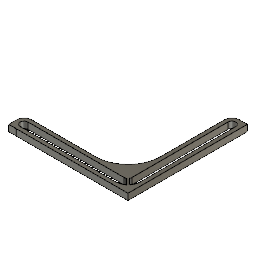
lidar_camera_frontplate v1 (Autodesk Fusion 360 archive; units mm, degrees)
design "front_L"
Autodesk Fusion 360 part; units mm, degrees
note: some values were not read from the file. Chosen so that the rebuilt part matches the saved one: that a step has no effect. Set by a fixed rule: which sketch regions a step uses.
sketch "Sketch1" plane through (0, 0, 0) normal (0, 0, 1) x (1, 0, 0)
  line L0 (20, 90) -> (17, 90)
  line L1 (17, 16) -> (17, 90)
  line L2 (23, 90) -> (23, 16)
  line L3 (-60, 7) -> (14, 7)
  line L4 (14, 13) -> (-60, 13)
  arc A0 (23, 90) -> (17, 89.9988) centre (20, 90) ccw
  arc A1 (-60, 13) -> (-60, 7) centre (-60, 10) ccw
  line L5 (-60, 4) -> (-66, 4)
  line L6 (-66, 4) -> (-66, 10)
  line L7 (-60, 16) -> (-11, 16)
  line L8 (14, 41) -> (14, 90)
  line L9 (20, 96) -> (26, 96)
  line L10 (26, 96) -> (26, 4)
  line L11 (26, 4) -> (-60, 4)
  arc A2 (-60, 16) -> (-66, 10) centre (-60, 10) ccw
  arc A3 (-11, 16) -> (14, 41) centre (-11, 41) ccw
  arc A4 (20, 96) -> (14, 90) centre (20, 90) ccw
  line L12 (18, 13) -> (16.823, 14.177)
  line L13 (18, 13) -> (20.4495, 10.5505)
  line L14 (17, 12) -> (15.823, 13.177)
  line L15 (17, 12) -> (19.8443, 9.1557)
  arc A5 (14, 13) -> (15.2595, 13.2772) centre (14, 16) ccw
  arc A6 (16.7228, 14.7405) -> (17, 16) centre (14, 16) ccw
  arc A7 (14, 7) -> (19.8443, 9.1557) centre (14, 16) ccw
  arc A8 (21.2032, 10.6043) -> (23, 16) centre (14, 16) ccw
  arc A9 (15.823, 13.177) -> (15.2595, 13.2772) centre (15.4695, 12.8234) ccw
  arc A10 (16.7228, 14.7405) -> (16.823, 14.177) centre (17.1766, 14.5305) ccw
  arc A11 (20.4495, 10.5505) -> (21.2032, 10.6043) centre (20.803, 10.9041) ccw
  dimension "d1" = 6
  dimension "d4" = 6
  dimension "d6" = 3
  dimension "d7" = 9
  dimension "d8" = 3
  dimension "d9" = 6
  dimension "d10" = 25
  dimension "d11" = 6
  dimension "d13" = 92
  dimension "d14" = 92
  dimension "d15" = 12
  dimension "d16" = 0.5
  constraint coincident L0.start A0.centre
  constraint coincident L0.end A0
  constraint horizontal L0
  constraint perpendicular L0 L1
  constraint tangent L4 A1
  constraint coincident L1 A0.end
  constraint tangent L1 A5
  constraint tangent L4 A5
  constraint horizontal L3
  constraint tangent L2 A7
  constraint tangent L3 A7
  constraint perpendicular L5 L6
  constraint perpendicular L7 L8
  constraint perpendicular L8 L9
  constraint perpendicular L9 L10
  constraint tangent L6 A2
  constraint tangent L7 A2
  constraint tangent L8 A3
  constraint tangent L7 A3
  constraint tangent L9 A4
  constraint tangent L8 A4
  constraint concentric A5 A6
  constraint concentric A7 A8
  constraint tangent L14 A9
  constraint tangent A5 A9
  constraint tangent L12 A10
  constraint tangent A6 A10
  constraint equal A9 A10
  constraint tangent L13 A11
  constraint tangent A8 A11
  constraint equal A9 A11
  measures "d1" diameter of A0
  measures "d4" diameter of A1
  measures "d6" radius of A5
  measures "d7" radius of A7
  measures "d8" distance of L3.start L5.start
  measures "d9" radius of A2
  measures "d10" radius of A3
  measures "d11" radius of A4
  measures "d13" distance of L9.end L10.end
  measures "d14" distance of L5.end L10.end
  measures "d15" distance of L7 L11
  measures "d16" radius of A9
extrude "Extrude1" add sketch "Sketch1" along normal blind 5

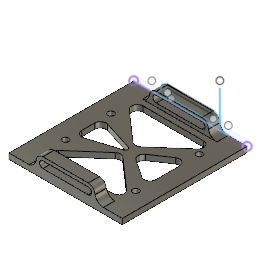
design "lidar_holder"
Autodesk Fusion 360 part; units mm, degrees
sketch "Sketch1" plane through (0, 0, 0) normal (0, 0, 1) x (1, 0, 0)
  line L0 (0, 0) -> (100, 0)
  line L1 (100, 0) -> (100, 110)
  line L2 (100, 110) -> (0, 110)
  line L3 (0, 110) -> (0, 0)
  circle A0 centre (15, 35) radius 2.75
  circle A1 centre (15, 75) radius 2.75
  circle A2 centre (85, 83) radius 2.75
  circle A3 centre (85, 27) radius 2.75
  line L4 (85, 35) -> (85, 75)
  line L5 (15, 67.5) -> (15, 42.5)
  line L6 (85, 35) -> (55, 55)
  line L7 (85, 75) -> (55, 55)
  line L8 (50, 50) -> (10, 15)
  line L9 (10, 15) -> (90, 15)
  line L10 (90, 15) -> (50, 50)
  line L11 (50, 60) -> (90, 95)
  line L12 (90, 95) -> (10, 95)
  line L13 (10, 95) -> (50, 60)
  line L14 (15, 42.5) -> (54.5, 55)
  line L15 (54.5, 55) -> (15, 67.5)
  dimension "d1" = 5.5
  dimension "d2" = 5.5
  dimension "d3" = 5.5
  dimension "d4" = 5.5
  dimension "d5" = 40
  dimension "d6" = 56
  dimension "d7" = 70
  dimension "d9" = 100
  dimension "d10" = 110
  dimension "d11" = 27
  dimension "d12" = 15
  dimension "d63" = 15
  dimension "d66" = 15
  dimension "d67" = 7.5
  dimension "d68" = 7.5
  dimension "d72" = 15
  dimension "d73" = 15
  dimension "d76" = 50
  dimension "d77" = 10
  dimension "d78" = 10
  dimension "d80" = 56.31
  dimension "d81" = 56.31
  dimension "d140" = 10
  dimension "d141" = 41.186
  dimension "d142" = 41.186
  dimension "d143" = 72.44
  dimension "d152" = 35
  dimension "d153" = 35
  dimension "d154" = 35
  constraint horizontal L0
  constraint vertical L1
  constraint horizontal L2
  constraint vertical L3
  constraint coincident L0.start L3.end
  constraint vertical A0.centre A1.centre
  constraint vertical A2.centre A3.centre
  constraint vertical L4
  constraint vertical L5
  constraint horizontal L9
  constraint parallel L8 L11
  constraint parallel L10 L13
  constraint horizontal L6.end L14.end
  measures "d1" diameter of A0
  measures "d2" diameter of A1
  measures "d3" diameter of A2
  measures "d4" diameter of A3
  measures "d5" vertical distance of A0.centre A1.centre
  measures "d6" vertical distance of A2.centre A3.centre
  measures "d7" horizontal distance of A1.centre A2.centre
  measures "d9" distance of L1.end L2.end
  measures "d10" distance of L0.end L1.end
  measures "d11" distance of L2 A2.centre
  measures "d12" distance of L1 A3.centre
  measures "d63" distance of L1 L4
  measures "d66" distance of L3 L5
  measures "d67" distance of A0.centre L5.end
  measures "d68" distance of A1.centre L5.start
  measures "d72" distance of L0 L9
  measures "d73" distance of L2 L12
  measures "d76" distance of L2 L11.start
  measures "d77" distance of L3 L12.end
  measures "d78" distance of L3 L8.end
  measures "d80" angle of L4 L6
  measures "d81" angle of L4 L7
  measures "d140" distance of L1 L9.end
  measures "d141" angle of L12 L13
  measures "d142" angle of L11 L12
  measures "d143" angle of L5 L14
  measures "d152" distance of L2 L4.end
  measures "d153" distance of L0 L4.start
  measures "d154" distance of L2 A1.centre
extrude "Extrude13" add sketch "Sketch1" along normal blind 5
sketch "Sketch2" plane through (0, 110, 0) normal (0, 1, 0) x (-1, 0, 0)
  line L0 (-100, 0) -> (0, 0)
  line L1 (0, 0) -> (0, 10)
  line L2 (0, 10) -> (-100, 10)
  line L3 (-100, 10) -> (-100, 0)
  arc A0 (-29.9676, 8) -> (-29.9676, 14) centre (-29.9676, 11) ccw
  line L4 (-75.9121, 43) -> (-76, 43)
  line L5 (-29.9676, 8) -> (-33.1608, 8)
  line L6 (-29.9676, 14) -> (-69.9676, 14)
  line L7 (-69.9676, 8) -> (-29.9676, 8)
  arc A1 (-69.9676, 17) -> (-75.9676, 11) centre (-69.9676, 11) ccw
  line L8 (-69.9676, 17) -> (-29.9676, 17)
  line L9 (-76, 37.0055) -> (-75.9676, 11)
  arc A2 (-69.9676, 14) -> (-69.9676, 8) centre (-69.9676, 11) ccw
  arc A3 (-23.9676, 11) -> (-29.9676, 17) centre (-29.9676, 11) ccw
  line L10 (-23.9676, 5) -> (-75.9676, 5)
  line L11 (-75.9676, 5) -> (-83.3383, 5)
  line L12 (-23.9676, 5) -> (-17.9511, 5)
  arc A4 (-83.3383, 5) -> (-75.9676, 11) centre (-83.3383, 12.5273) ccw
  arc A5 (-23.9676, 11) -> (-17.9511, 5) centre (-16.0025, 12.9705) ccw
  line L13 (0, 5) -> (-100, 5)
  dimension "d108" = 6
  dimension "d109" = 6
  dimension "d110" = 3
  dimension "d111" = 40
  dimension "d112" = 6
  dimension "d115" = 6
  dimension "d116" = 40
  dimension "d119" = 6
  dimension "d120" = 52
  dimension "d121" = 3
  dimension "d135" = 12
  constraint tangent L6 A2
  constraint horizontal L6
  constraint horizontal L8
  constraint parallel L4 L8
  constraint concentric A1 A2
  constraint tangent A1 L9
  constraint coincident L8.start A1
  constraint coincident L9.start A1
  constraint coincident A1.start L8
  constraint concentric A0 A3
  constraint tangent L11 A4
  constraint horizontal L10
  measures "d108" diameter of A2
  measures "d109" diameter of A0
  measures "d110" distance of L6 L8
  measures "d111" distance of A0.end L6.end
  measures "d112" distance of A1.centre L9
  measures "d115" radius of A3
  measures "d116" distance of A1.centre A0.centre
  measures "d119" distance of A3.start L10.start
  measures "d120" distance of L10.start L10.end
  measures "d121" distance of L7 L10
  measures "d135" distance of L8 L13
extrude "Extrude14" add sketch "Sketch2" against normal blind 110 contours L2 A0 L5 L7 A2 L10 L11 L12 A4 A5 L13 | L2 A0 L6 A1 L8 A2 A3 A4 A5
sketch "Sketch6" plane through (0, 0, 22) normal (0, 0, 1) x (-1, 0, 0)
  line L0 (-70.0055, -110) -> (-30, -110)
  line L1 (-30, -110) -> (-30, 0)
  line L2 (-30, 0) -> (-70.0055, 0)
  line L3 (-70.0055, 0) -> (-70.0055, -110)
  line L4 (-10, -10) -> (-90, -10)
  line L5 (-90, -10) -> (-90, -100)
  line L6 (-90, -100) -> (-10, -100)
  line L7 (-10, -100) -> (-10, -10)
  line L8 (-69.9676, -110) -> (-29.9676, -110)
  line L9 (-100, 0) -> (-100, -110)
  line L10 (0, -110) -> (0, 0)
  dimension "d127" = 10
  dimension "d128" = 10
  dimension "d129" = 10
  dimension "d130" = 10
  constraint horizontal L4
  constraint vertical L5
  constraint horizontal L6
  constraint vertical L7
  measures "d127" distance of L6 L8
  measures "d128" distance of L2 L4
  measures "d129" distance of L5 L9
  measures "d130" distance of L7 L10
extrude "Extrude15" cut sketch "Sketch6" against normal blind 17 contours L3 L4 L5 L6 | L1 L3 L4 L6 | L1 L4 L6 L7
fillet "Fillet4" radius 2 1 edges at (54.5, 55, 2.5)
fillet "Fillet5" radius 5 3 edges at (50, 50, 2.5) (55, 55, 2.5) (50, 60, 2.5)
fillet "Fillet6" radius 5 6 edges at (10, 15, 2.5) (90, 15, 2.5) (85, 35, 2.5) (85, 75, 2.5) (90, 95, 2.5) (10, 95, 2.5)
fillet "Fillet7" radius 5 2 edges at (15, 67.5, 2.5) (15, 42.5, 2.5)

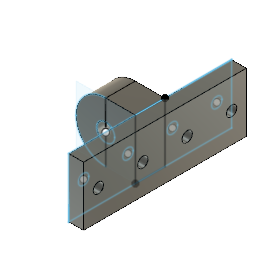
design "camera_joint_male"
Autodesk Fusion 360 part; units mm, degrees
ref_plane "WorkPlane1" through (-98.2453, -42.8288, 162.8804) normal (-0.999826, -0.005173, -0.017916) x (-0.018434, 0.129368, 0.991425)
pattern_linear "R-Pattern1" [no effect]
extrude "Extrude9" [no effect]
extrude "Extrude10" [no effect]
sketch "Sketch12" plane through (-95.5151, -0.4942, -1.7115) normal (-0.999826, -0.005173, -0.017916) x (0.005174, -0.999987, 0)
sketch "Sketch13" plane through (0.6338, -122.4984, 0) normal (0.005174, -0.999987, 0) x (0.999987, 0.005174, 0)
extrude "Extrude15" [no effect]
sketch "Sketch16" plane through (0, 0, 0) normal (1, 0, 0) x (0, 1, 0)
  line L0 (10, 50) -> (65, 50)
  line L1 (65, 50) -> (65, 30)
  line L2 (65, 30) -> (10, 30)
  line L3 (10, 30) -> (10, 50)
  circle A0 centre (45, 40) radius 1.75
  circle A1 centre (60, 40) radius 1.75
  circle A2 centre (30, 40) radius 1.75
  circle A3 centre (15, 40) radius 1.75
  dimension "d55" = 55
  dimension "d56" = 20
  dimension "d60" = 3.5
  dimension "d61" = 3.5
  dimension "d62" = 15
  dimension "d63" = 3.5
  dimension "d64" = 3.5
  dimension "d66" = 15
  dimension "d67" = 5
  dimension "d68" = 15
  dimension "d69" = 10
  constraint horizontal L0
  constraint vertical L1
  constraint horizontal L2
  constraint vertical L3
  constraint horizontal A2.centre A3.centre
  measures "d55" distance of L0.start L0.end
  measures "d56" distance of L0.end L1.end
  measures "d60" diameter of A1
  measures "d61" diameter of A0
  measures "d62" distance of A1.centre A0.centre
  measures "d63" diameter of A3
  measures "d64" diameter of A2
  measures "d66" horizontal distance of A2.centre A3.centre
  measures "d67" distance of L1 A1.centre
  measures "d68" distance of A0.centre A2.centre
  measures "d69" distance of L0 A1.centre
extrude "Extrude16" add sketch "Sketch16" along normal blind 5
sketch "Sketch17" plane through (0, 0, 0) normal (-1, 0, 0) x (0, -1, 0)
  circle A0 centre (-45, 40) radius 1.75
  circle A1 centre (-30, 40) radius 1.75
  circle A2 centre (-15, 40) radius 1.75
  circle A3 centre (-60, 40) radius 1.75
  line L0 (-65, 30) -> (-10, 30)
  line L1 (-10, 30) -> (-10, 50)
  line L2 (-10, 50) -> (-65, 50)
  line L3 (-65, 50) -> (-65, 30)
  line L4 (-42.5, 50) -> (-32.5, 50)
  line L5 (-32.5, 50) -> (-32.5, 30)
  line L6 (-32.5, 30) -> (-42.5, 30)
  line L7 (-42.5, 30) -> (-42.5, 50)
  dimension "d72" = 10
  dimension "d73" = 2.5
  constraint horizontal L4
  constraint vertical L5
  constraint horizontal L6
  constraint vertical L7
  constraint coincident L0 L5.end
  constraint coincident L2 L4.start
  measures "d72" distance of L4.start L4.end
  measures "d73" horizontal distance of A0.centre L4.start
extrude "Extrude17" add sketch "Sketch17" along normal blind 20 contours L0 L2 L4 L5 L6 L7
sketch "Sketch18" plane through (0, 32.5, 0) normal (0, -1, 0) x (1, 0, 0)
  line L0 (0, 30) -> (0, 50)
  line L1 (0, 50) -> (-20, 50)
  line L2 (-20, 50) -> (-20, 30)
  line L3 (-20, 30) -> (0, 30)
  line L4 (-10, 50) -> (-10, 30)
  arc A0 (-10, 50) -> (-20, 40) centre (-10, 40) ccw
  arc A1 (-20, 40) -> (-10, 30) centre (-10, 40) ccw
  circle A2 centre (-10, 40) radius 3
  dimension "d76" = 10
  dimension "d77" = 10
  dimension "d78" = 6
  constraint vertical L4
  constraint midpoint L3 L4.end
  constraint coincident L4.start A0.start
  constraint coincident A0.end A1.start
  constraint coincident L4.end A1.end
  constraint concentric A1 A2
  measures "d76" radius of A0
  measures "d77" radius of A1
  measures "d78" diameter of A2
extrude "Extrude18" cut sketch "Sketch18" against normal blind 10 contours L2 L3 A1 | L1 L2 A0 | L4 A2 | L4 A2

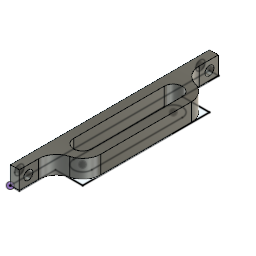
design "front_I"
Autodesk Fusion 360 part; units mm, degrees
sketch "Sketch1" plane through (0, 0, 0) normal (0, 0, 1) x (1, 0, 0)
  line L0 (0, 0) -> (0, 66)
  line L1 (0, 66) -> (3, 66)
  line L2 (3, 66) -> (3, 54)
  line L3 (0, 0) -> (3, 0)
  line L4 (3, 0) -> (3, 12)
  line L5 (3, 12) -> (12, 12)
  line L6 (12, 54) -> (12, 12)
  line L7 (3, 54) -> (12, 54)
  line L8 (9, 18) -> (9, 48)
  line L9 (3, 18) -> (3, 48)
  arc A0 (9, 48) -> (3, 48) centre (6, 48) ccw
  arc A1 (3, 18) -> (9, 18) centre (6, 18) ccw
  dimension "d1" = 3
  dimension "d5" = 3
  dimension "d6" = 12
  dimension "d7" = 9
  dimension "d13" = 9
  dimension "d14" = 12
  dimension "d18" = 66
  dimension "d20" = 6
  dimension "d21" = 6
  dimension "d22" = 6
  dimension "d23" = 6
  dimension "d24" = 6
  dimension "d25" = 6
  constraint coincident L0.start L3.start
  constraint vertical L0
  constraint perpendicular L0 L1
  constraint perpendicular L1 L2
  constraint perpendicular L0 L3
  constraint perpendicular L3 L4
  constraint perpendicular L4 L5
  constraint perpendicular L6 L7
  constraint tangent L8 A0
  constraint tangent L9 A0
  measures "d1" distance of L0.end L1.end
  measures "d5" distance of L0.start L3.end
  measures "d6" distance of L3.end L4.end
  measures "d7" distance of L4.end L5.end
  measures "d13" distance of L2.end L6.start
  measures "d14" distance of L1 L7
  measures "d18" distance of L0.start L0.end
  measures "d20" diameter of A0
  measures "d21" distance of L7 A0.centre
  measures "d22" distance of L0 A0.centre
  measures "d23" diameter of A1
  measures "d24" distance of L6 A1.centre
  measures "d25" distance of L5 A1.centre
extrude "Extrude2" add sketch "Sketch1" along normal blind 6
sketch "Sketch2" plane through (0, 0, 0) normal (-1, 0, 0) x (0, -1, 0)
  line L0 (-66, 0) -> (0, 0)
  line L1 (0, 0) -> (0, 6)
  line L2 (0, 6) -> (-66, 6)
  line L3 (-66, 6) -> (-66, 0)
  circle A0 centre (-3, 3) radius 1.5
  circle A1 centre (-63, 3) radius 1.5
  dimension "d34" = 3
  dimension "d35" = 3
  dimension "d36" = 3
  dimension "d37" = 3
  dimension "d38" = 3
  dimension "d44" = 60
  measures "d34" diameter of A0
  measures "d35" distance of L2 A0.centre
  measures "d36" distance of L1 A0.centre
  measures "d37" diameter of A1
  measures "d38" distance of L2 A1.centre
  measures "d44" distance of A0.centre A1.centre
extrude "Extrude3" cut sketch "Sketch2" against normal blind 10 contours A0 | A1
fillet "Fillet3" radius 6 4 edges at (12, 12, 3) (12, 54, 3) (3, 54, 3) (3, 12, 3)
equation "d18 = 60 mm + 6 mm"
equation "d44 = ( 15 * 4 ) * 1 mm"
